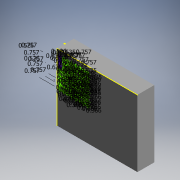
# Autodesk Inventor part: thermocylcer block
Saved by Autodesk Inventor 2018 (Build 220112000, 112)
## iProperties
Part Number: thermocylcer block
Material: Generic
Document SubType Name: Modeling
Designer: Intel
Appearance: Generic
Author: Intel
Autodesk Inventor part; units mm, degrees
ref_plane "YZ Plane" through (0, 0, 0) normal (1, 0, 0) x (0, 1, 0)
ref_plane "XZ Plane" through (0, 0, 0) normal (0, 1, 0) x (-1, 0, 0)
ref_plane "XY Plane" through (0, 0, 0) normal (0, 0, 1) x (1, 0, 0)
sketch "Sketch1" plane through (0, 0, 0) normal (0, 0, 1) x (1, 0, 0)
  line L0 (0, 0) -> (153.162, 0)
  line L1 (153.162, 0) -> (153.162, -127.254)
  line L2 (153.162, -127.254) -> (0, -127.254)
  line L3 (0, -127.254) -> (0, 0)
  dimension "d0" = 153.162
  dimension "d1" = 127.254
  constraints: 8 end point, 2 parallel, 1 horizontal, 1 perpendicular
  measures "d0" distance of L1.end L2.end
  measures "d1" distance of L0.end L1.end
extrude "Extrusion1" add sketch "Sketch1" along normal blind 32.004
sketch "Sketch2" plane through (0, 0, 32.004) normal (0, 0, 1) x (1, 0, 0)
  line L0 (0, 0) -> (0, -127.254) projected
  line L1 (153.162, 0) -> (0, 0) projected
  circle A0 centre (5.2578, -64.6557) radius 1.8288
  circle A1 centre (5.2578, -57.0865) radius 1.8288
  circle A2 centre (12.827, -57.0865) radius 1.8288
  circle A3 centre (12.827, -64.6557) radius 1.8288
  circle A4 centre (12.827, -49.5173) radius 1.8288
  circle A5 centre (5.2578, -49.5173) radius 1.8288
  circle A6 centre (12.827, -41.9481) radius 1.8288
  circle A7 centre (5.2578, -41.9481) radius 1.8288
  circle A8 centre (20.3962, -64.6557) radius 1.8288
  circle A9 centre (20.3962, -57.0865) radius 1.8288
  circle A10 centre (20.3962, -49.5173) radius 1.8288
  circle A11 centre (5.2578, -34.3789) radius 1.8288
  circle A12 centre (12.827, -34.3789) radius 1.8288
  circle A13 centre (12.827, -26.8097) radius 1.8288
  circle A14 centre (12.827, -19.2405) radius 1.8288
  circle A15 centre (5.26, -19.2405) radius 1.8288
  circle A16 centre (5.2578, -26.8097) radius 1.8288
  circle A17 centre (27.9654, -64.6557) radius 1.8288
  circle A18 centre (27.9654, -57.0865) radius 1.8288
  circle A19 centre (27.9654, -49.5173) radius 1.8288
  circle A20 centre (27.9654, -41.9481) radius 1.8288
  circle A21 centre (27.9654, -34.3789) radius 1.8288
  circle A22 centre (27.9654, -26.8097) radius 1.8288
  circle A23 centre (35.5346, -64.6557) radius 1.8288
  circle A24 centre (35.5346, -57.0865) radius 1.8288
  circle A25 centre (35.5346, -49.5173) radius 1.8288
  circle A26 centre (35.5346, -41.9481) radius 1.8288
  circle A27 centre (35.5346, -34.3789) radius 1.8288
  circle A28 centre (35.5346, -26.8097) radius 1.8288
  circle A29 centre (35.5346, -19.2405) radius 1.8288
  circle A30 centre (27.9654, -19.2405) radius 1.8288
  circle A31 centre (20.3962, -19.2405) radius 1.8288
  circle A32 centre (20.3962, -26.8097) radius 1.8288
  circle A33 centre (20.3962, -34.3789) radius 1.8288
  circle A34 centre (20.3962, -11.6713) radius 1.8288
  circle A35 centre (27.9654, -11.6713) radius 1.8288
  circle A36 centre (35.5346, -11.6713) radius 1.8288
  circle A37 centre (43.1038, -11.6713) radius 1.8288
  circle A38 centre (43.1038, -19.2405) radius 1.8288
  circle A39 centre (43.1038, -26.8097) radius 1.8288
  circle A40 centre (43.1038, -34.3789) radius 1.8288
  circle A41 centre (43.1038, -41.9481) radius 1.8288
  circle A42 centre (43.1038, -49.5173) radius 1.8288
  circle A43 centre (43.1038, -57.0865) radius 1.8288
  circle A44 centre (43.1038, -64.6557) radius 1.8288
  circle A45 centre (50.673, -64.6557) radius 1.8288
  circle A46 centre (58.2422, -64.6557) radius 1.8288
  circle A47 centre (50.673, -57.0865) radius 1.8288
  circle A48 centre (58.2422, -57.0865) radius 1.8288
  circle A49 centre (50.673, -49.5173) radius 1.8288
  circle A50 centre (58.2422, -49.5173) radius 1.8288
  circle A51 centre (58.2422, -41.9481) radius 1.8288
  circle A52 centre (50.673, -41.9481) radius 1.8288
  circle A53 centre (50.673, -34.3789) radius 1.8288
  circle A54 centre (58.2422, -34.3789) radius 1.8288
  circle A55 centre (58.2422, -26.8097) radius 1.8288
  circle A56 centre (50.673, -26.8097) radius 1.8288
  circle A57 centre (50.673, -19.2405) radius 1.8288
  circle A58 centre (58.2422, -19.2405) radius 1.8288
  circle A59 centre (58.2422, -11.6713) radius 1.8288
  circle A60 centre (50.673, -11.6713) radius 1.8288
  circle A61 centre (5.2578, -26.8097) radius 1.8288
  circle A62 centre (5.2578, -11.6713) radius 1.8288
  circle A63 centre (12.827, -11.6713) radius 1.8288
  circle A64 centre (20.3962, -41.9481) radius 1.8288
  circle A65 centre (5.2578, -64.6557) radius 3.175
  circle A66 centre (5.2578, -57.0865) radius 3.175
  circle A67 centre (5.2578, -49.5173) radius 3.175
  circle A68 centre (12.827, -64.6557) radius 3.175
  circle A69 centre (12.827, -57.0865) radius 3.175
  circle A70 centre (12.827, -49.5173) radius 3.175
  circle A71 centre (12.827, -41.9481) radius 3.175
  circle A72 centre (5.2578, -41.9481) radius 3.175
  circle A73 centre (5.2578, -34.3789) radius 3.175
  circle A74 centre (12.827, -34.3789) radius 3.175
  circle A75 centre (20.3962, -64.6557) radius 3.175
  circle A76 centre (20.3962, -57.0865) radius 3.175
  circle A77 centre (20.3962, -49.5173) radius 3.175
  circle A78 centre (20.3962, -41.9481) radius 3.175
  circle A79 centre (20.3962, -34.3789) radius 3.175
  circle A80 centre (20.3962, -26.8097) radius 3.175
  circle A81 centre (12.827, -26.8097) radius 3.175
  circle A82 centre (5.2578, -26.8097) radius 3.175
  circle A83 centre (27.9654, -64.6557) radius 3.175
  circle A84 centre (27.9654, -57.0865) radius 3.175
  circle A85 centre (27.9654, -49.5173) radius 3.175
  circle A86 centre (27.9654, -41.9481) radius 3.175
  circle A87 centre (27.9654, -34.3789) radius 3.175
  circle A88 centre (27.9654, -26.8097) radius 3.175
  circle A89 centre (35.5346, -64.6557) radius 3.175
  circle A90 centre (35.5346, -57.0865) radius 3.175
  circle A91 centre (35.5346, -49.5173) radius 3.175
  circle A92 centre (35.5346, -41.9481) radius 3.175
  circle A93 centre (35.5346, -34.3789) radius 3.175
  circle A94 centre (35.5346, -26.8097) radius 3.175
  circle A95 centre (43.1038, -34.3789) radius 3.175
  circle A96 centre (43.1038, -41.9481) radius 3.175
  circle A97 centre (43.1038, -26.8097) radius 3.175
  circle A98 centre (43.1038, -49.5173) radius 3.175
  circle A99 centre (43.1038, -57.0865) radius 3.175
  circle A100 centre (43.1038, -64.6557) radius 3.175
  circle A101 centre (50.673, -64.6557) radius 3.175
  circle A102 centre (50.673, -57.0865) radius 3.175
  circle A103 centre (50.673, -49.5173) radius 3.175
  circle A104 centre (50.673, -41.9481) radius 3.175
  circle A105 centre (50.673, -34.3789) radius 3.175
  circle A106 centre (58.2422, -64.6557) radius 3.175
  circle A107 centre (58.2422, -57.0865) radius 3.175
  circle A108 centre (58.2422, -49.5173) radius 3.175
  circle A109 centre (58.2422, -41.9481) radius 3.175
  circle A110 centre (58.2422, -34.3789) radius 3.175
  circle A111 centre (58.2422, -26.8097) radius 3.175
  circle A112 centre (50.673, -26.8097) radius 3.175
  circle A113 centre (58.2422, -19.2405) radius 3.175
  circle A114 centre (50.673, -19.2405) radius 3.175
  circle A115 centre (43.1038, -19.2405) radius 3.175
  circle A116 centre (35.5346, -19.2405) radius 3.175
  circle A117 centre (27.9654, -19.2405) radius 3.175
  circle A118 centre (20.3962, -19.2405) radius 3.175
  circle A119 centre (12.827, -19.2405) radius 3.175
  circle A120 centre (5.26, -19.2405) radius 3.175
  circle A121 centre (5.2578, -11.6713) radius 3.175
  circle A122 centre (12.827, -11.6713) radius 3.175
  circle A123 centre (20.3962, -11.6713) radius 3.175
  circle A124 centre (27.9654, -11.6713) radius 3.175
  circle A125 centre (35.5346, -11.6713) radius 3.175
  circle A126 centre (43.1038, -11.6713) radius 3.175
  circle A127 centre (50.673, -11.6713) radius 3.175
  circle A128 centre (58.2422, -11.6713) radius 3.175
  dimension "d4" = 5.2578
  dimension "d5" = 11.6713
  dimension "d6" = 7.5692
  dimension "d7" = 5.26
  dimension "d8" = 7.5692
  dimension "d9" = 5.2578
  dimension "d10" = 7.5692
  dimension "d11" = 7.5692
  dimension "d12" = 5.2578
  dimension "d13" = 7.5692
  dimension "d14" = 7.5692
  dimension "d15" = 7.5692
  dimension "d16" = 7.5692
  dimension "d17" = 7.5692
  dimension "d18" = 7.5692
  dimension "d19" = 7.5692
  dimension "d20" = 7.5692
  dimension "d21" = 7.5692
  dimension "d22" = 7.5692
  dimension "d23" = 3.6576
  dimension "d26" = 3.6576
  dimension "d27" = 3.6576
  dimension "d28" = 3.6576
  dimension "d29" = 3.6576
  dimension "d30" = 3.6576
  dimension "d31" = 3.6576
  dimension "d32" = 3.6576
  dimension "d33" = 3.6576
  dimension "d34" = 3.6576
  dimension "d35" = 3.6576
  dimension "d36" = 3.6576
  dimension "d37" = 3.6576
  dimension "d38" = 3.6576
  dimension "d39" = 3.6576
  dimension "d40" = 3.6576
  dimension "d41" = 3.6576
  dimension "d42" = 3.6576
  dimension "d43" = 3.6576
  dimension "d44" = 3.6576
  dimension "d45" = 3.6576
  dimension "d46" = 3.6576
  dimension "d47" = 3.6576
  dimension "d48" = 3.6576
  dimension "d49" = 3.6576
  dimension "d50" = 3.6576
  dimension "d51" = 3.6576
  dimension "d52" = 3.6576
  dimension "d53" = 3.6576
  dimension "d54" = 3.6576
  dimension "d55" = 3.6576
  dimension "d56" = 3.6576
  dimension "d57" = 3.6576
  dimension "d58" = 3.6576
  dimension "d59" = 3.6576
  dimension "d60" = 3.6576
  dimension "d61" = 3.6576
  dimension "d62" = 3.6576
  dimension "d63" = 3.6576
  dimension "d64" = 3.6576
  dimension "d65" = 3.6576
  dimension "d66" = 3.6576
  dimension "d67" = 3.6576
  dimension "d68" = 3.6576
  dimension "d69" = 3.6576
  constraints: 129 centre point, 129 coincident
  measures "d4" distance from line of L0 point (5.258, -11.671)
  measures "d5" distance from line of point (5.258, -11.671) L1
  measures "d6" distance of point (5.258, -11.671) point (5.26, -19.24)
  measures "d7" distance from line of L0 point (5.26, -19.24)
  measures "d8" distance of point (5.258, -26.81) point (5.26, -19.24)
  measures "d9" distance from line of L0 point (5.258, -26.81)
  measures "d10" distance of point (5.258, -26.81) point (5.258, -34.379)
  measures "d11" distance of point (5.258, -41.948) point (5.258, -34.379)
  measures "d12" distance from line of L0 point (5.258, -41.948)
  measures "d13" distance of point (5.258, -49.517) point (5.258, -41.948)
  measures "d14" distance of point (5.258, -57.086) point (5.258, -49.517)
  measures "d15" distance of point (5.258, -64.656) point (5.258, -57.086)
  measures "d16" distance of point (5.258, -64.656) point (12.827, -64.656)
  measures "d17" distance of point (12.827, -64.656) point (20.396, -64.656)
  measures "d18" distance of point (20.396, -64.656) point (27.965, -64.656)
  measures "d19" distance of point (27.965, -64.656) point (35.535, -64.656)
  measures "d20" distance of point (35.535, -64.656) point (43.104, -64.656)
  measures "d21" distance of point (43.104, -64.656) point (50.673, -64.656)
  measures "d22" distance of point (50.673, -64.656) point (58.242, -64.656)
  measures "d23" diameter of A0
  measures "d26" diameter of A1
  measures "d27" diameter of A2
  measures "d28" diameter of A3
  measures "d29" diameter of A4
  measures "d30" diameter of A5
  measures "d31" diameter of A6
  measures "d32" diameter of A7
  measures "d33" diameter of A8
  measures "d34" diameter of A9
  measures "d35" diameter of A10
  measures "d36" diameter of A11
  measures "d37" diameter of A12
  measures "d38" diameter of A13
  measures "d39" diameter of A14
  measures "d40" diameter of A15
  measures "d41" diameter of A16
  measures "d42" diameter of A17
  measures "d43" diameter of A18
  measures "d44" diameter of A19
  measures "d45" diameter of A20
  measures "d46" diameter of A21
  measures "d47" diameter of A22
  measures "d48" diameter of A23
  measures "d49" diameter of A24
  measures "d50" diameter of A25
  measures "d51" diameter of A26
  measures "d52" diameter of A27
  measures "d53" diameter of A28
  measures "d54" diameter of A29
  measures "d55" diameter of A30
  measures "d56" diameter of A31
  measures "d57" diameter of A32
  measures "d58" diameter of A33
  measures "d59" diameter of A34
  measures "d60" diameter of A35
  measures "d61" diameter of A36
  measures "d62" diameter of A37
  measures "d63" diameter of A38
  measures "d64" diameter of A39
  measures "d65" diameter of A40
  measures "d66" diameter of A41
  measures "d67" diameter of A42
  measures "d68" diameter of A43
  measures "d69" diameter of A44
extrude "Extrusion2" cut sketch "Sketch2" against normal blind 14.6558 contours A0
extrude "Extrusion3" cut sketch "Sketch2" against normal blind 14.6558 contours A0 | A1 | A2 | A3 | A4 | A5 | A6 | A7 | A8 | A9 | A10 | A11 | A12 | A13 | A14 | A15 | A16 | A17 | A18 | A19 | A20 | A21 | A22 | A23 | A24 | A25 | A26 | A27 | A28 | A29 | A30 | A31 | A32 | A33 | A34 | A35 | A36 | A37 | A38 | A39 | A40 | A41 | A42 | A43 | A44 | A45 | A46 | A47 | A48 | A49 | A50 | A51 | A52 | A53 | A54 | A55 | A56 | A57 | A58 | A59 | A60 | A62 | A63 | A64
sketch "Sketch3" plane through (12.827, -49.5173, 17.3482) normal (0, 0, 1) x (1, 0, 0)
  circle A0 centre (-6.5853, 36.1219) radius 5.8342
  circle A1 centre (-7.5692, 37.846) radius 1.8288 projected
  circle A2 centre (-7.5692, 37.846) radius 3.175
  point P0 (-12.827, 49.5173)
  dimension "d92" = 6.35
  constraints: 2 centre point, 1 coincident
  measures "d92" diameter of A2
body "Solid1"
